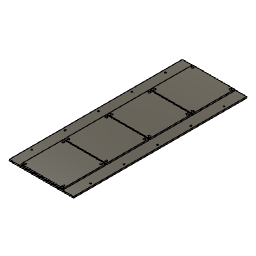
support_cartes_tlc v2 (Autodesk Fusion 360 design; units mm, degrees)
Autodesk Fusion 360 part; units mm, degrees
sketch "Esquisse1" plane through (0, 0, 0) normal (0, 0, 1) x (1, 0, 0)
  line L0 (0, 0) -> (152.5, 0)
  line L1 (152.5, 0) -> (152.5, 410)
  line L2 (152.5, 410) -> (0, 410)
  line L3 (0, 410) -> (0, 0)
  circle A0 centre (6.75, 47) radius 1.75
  line L4 (6.75, 47) -> (0, 47) construction
  line L5 (6.75, 47) -> (6.75, 0) construction
  circle A1 centre (145.75, 47) radius 1.75
  circle A2 centre (6.75, 126) radius 1.75
  circle A3 centre (145.75, 126) radius 1.75
  circle A4 centre (6.75, 205) radius 1.75
  circle A5 centre (145.75, 205) radius 1.75
  circle A6 centre (6.75, 284) radius 1.75
  circle A7 centre (145.75, 284) radius 1.75
  circle A8 centre (6.75, 363) radius 1.75
  circle A9 centre (145.75, 363) radius 1.75
  line L6 (145.75, 47) -> (152.5, 47) construction
  line L7 (6.75, 363) -> (6.75, 410) construction
  dimension "d2" = 6.75
  dimension "d3" = 3.5
  dimension "d33" = 139
  dimension "d34" = 316
  dimension "d40" = 410
  constraint horizontal L0
  constraint vertical L1
  constraint horizontal L2
  constraint vertical L3
  constraint coincident L0.start L3.end
  constraint coincident A0.centre L4.start
  constraint coincident L3 L4.end
  constraint perpendicular L3 L4
  constraint coincident L0 L5.end
  constraint perpendicular L0 L5
  constraint coincident A1.centre L6.start
  constraint coincident L1 L6.end
  constraint perpendicular L1 L6
  constraint equal L4 L6
  constraint coincident A8.centre L7.start
  constraint coincident L2 L7.end
  constraint perpendicular L2 L7
  constraint equal L5 L7
  measures "d2" distance of L3 A0.centre
  measures "d3" diameter of A0
  measures "d40" distance of L0 L2
extrude "Extrusion1" add sketch "Esquisse1" along normal blind 3 makes body 1
sketch "Esquisse2" plane through (0, 0, 3) normal (0, 0, 1) x (-1, 0, 0)
  circle A0 centre (-6.75, -47) radius 1.75
  line L0 (0, -410) -> (0, 0)
  line L1 (0, 0) -> (-152.5, 0)
  line L2 (-152.5, 0) -> (-152.5, -410)
  line L3 (-152.5, -410) -> (0, -410)
  line L4 (-26.25, -101.75) -> (-126.25, -101.75)
  line L5 (-126.25, -101.75) -> (-126.25, -1.75)
  line L6 (-126.25, -1.75) -> (-26.25, -1.75)
  line L7 (-26.25, -1.75) -> (-26.25, -101.75)
  line L8 (0, -67.3009) -> (-26.25, -67.3009) construction
  line L9 (-126.25, -67.3009) -> (-152.5, -67.3009) construction
  circle A1 centre (-145.75, -205) radius 1.75
  circle A2 centre (-6.75, -126) radius 1.75
  circle A3 centre (-6.75, -205) radius 1.75
  circle A4 centre (-145.75, -363) radius 1.75
  circle A5 centre (-6.75, -363) radius 1.75
  circle A6 centre (-145.75, -126) radius 1.75
  circle A7 centre (-6.75, -284) radius 1.75
  circle A8 centre (-145.75, -47) radius 1.75
  circle A9 centre (-145.75, -284) radius 1.75
  line L10 (-26.25, -101.75) -> (-126.25, -1.75) construction
  line L11 (-126.25, -101.75) -> (-26.25, -1.75) construction
  line L12 (-31.25, -96.75) -> (-121.25, -96.75) construction
  line L13 (-121.25, -96.75) -> (-121.25, -6.75) construction
  line L14 (-121.25, -6.75) -> (-31.25, -6.75) construction
  circle A10 centre (-31.25, -96.75) radius 2.5
  circle A11 centre (-121.25, -96.75) radius 2.5
  circle A12 centre (-121.25, -6.75) radius 2.5
  circle A13 centre (-31.25, -6.75) radius 2.5
  dimension "d27" = 100
  dimension "d28" = 100
  dimension "d42" = 90
  dimension "d43" = 5
  constraint horizontal L4
  constraint vertical L5
  constraint horizontal L6
  constraint vertical L7
  constraint coincident L0 L8.start
  constraint coincident L7 L8.end
  constraint perpendicular L7 L8
  constraint coincident L5 L9.start
  constraint coincident L2 L9.end
  constraint perpendicular L2 L9
  constraint equal L8 L9
  constraint coincident L5 L4.end
  constraint coincident L4 L5.start
  constraint coincident L10 L12.start
  constraint coincident L11 L12.end
  constraint perpendicular L7 L12
  constraint coincident L10 L13.end
  constraint perpendicular L12 L13
  constraint coincident L11 L14.end
  constraint perpendicular L13 L14
  constraint coincident L12.start A10.centre
  constraint coincident L12.end L13.start
  constraint coincident L13.end L14.start
  constraint coincident L14.end A13.centre
  constraint equal A10 A11
  constraint equal A10 A12
  constraint equal A10 A13
  measures "d27" distance of L4 L6
  measures "d28" distance of L5 L7
  measures "d42" distance of L12.start L12.end
  measures "d43" diameter of A10
extrude "Extrusion2" add sketch "Esquisse2" along normal blind 3 separate body contours L4 L5 L6 L7 makes body 2
pattern_linear "Réseau R1" count 1 spacing 0 along (1, 0, 0) count 4 spacing 102 along (0, 1, 0) of bodies 2 makes body 3 at (61.8609, 139.3168, 3) makes body 4 at (61.8609, 241.3168, 3) makes body 5 at (90.6391, 343.3168, 3)
hole "Perçage1" at (31.25, 6.75, 6) direction (0, 0, -1) diameter 3.5 depth 20 tip angle 180 bodies 1
hole "Perçage2" at (31.25, 96.75, 6) direction (0, 0, -1) diameter 3.5 depth 20 tip angle 180 bodies 1
pattern_linear "Réseau R2" count 4 spacing 102 along (0, 1, 0) count 2 spacing 90 along (1, 0, 0) of "Perçage1", "Perçage2"
equation "d2 = 5 mm + d3 / 2"
equation "d34 = ( 79 * 4 ) * 1 mm"
